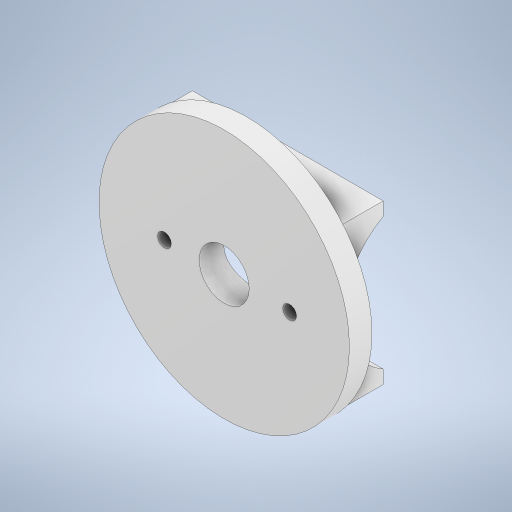
# Autodesk Inventor part: Hub Plate
Saved by Autodesk Inventor 2023 (Build 270158030, 158C)
## iProperties
Created: 2022-10-03
Part Number: Hub Plate
Material: ABS Plastic
Document SubType Name: Modeling
Designer: cjj5381
Density: 1.06 g/cm^3
Appearance: Smooth - White
Author: cjj5381
Autodesk Inventor part; units mm, degrees
ref_plane "YZ Plane" through (0, 0, 0) normal (1, 0, 0) x (0, 1, 0)
ref_plane "XZ Plane" through (0, 0, 0) normal (0, 1, 0) x (-1, 0, 0)
ref_plane "XY Plane" through (0, 0, 0) normal (0, 0, 1) x (1, 0, 0)
sketch "Sketch1" plane through (0, 0, 0) normal (1, 0, 0) x (0, 1, 0)
  circle A0 centre (0, -40) radius 30.1625 construction
  line L0 (31.75, 0) -> (-31.75, 0)
  line L1 (-31.75, 0) -> (-31.75, -25.4)
  line L2 (31.75, -25.4) -> (31.75, 0)
  line L3 (0, 0) -> (0, -115.458)
  arc A1 (26.3935, -25.4) -> (-26.3935, -25.4) centre (0, -40) ccw
  line L4 (-31.75, -25.4) -> (-26.3935, -25.4)
  line L5 (26.3935, -25.4) -> (31.75, -25.4)
  dimension "d1" = 60.325
  dimension "d3" = 63.5
  dimension "d4" = 40
  dimension "d5" = 25.4
  constraints: 12 end point, 4 point on circle, 3 parallel, 2 centre point, 1 concentric, 1 horizontal, 1 midpoint, 1 perpendicular, 1 point on line, 1 vertical, 1 vertical alignment, 1 other
  measures "d1" diameter of A0
  measures "d3" distance of L1.end L2.start
  measures "d4" distance from line of L0 A0.centre
  measures "d5" distance of L0.end L1.end
extrude "Extrusion1" add sketch "Sketch1" along normal mid plane 76.2
sketch "Sketch2" plane through (-38.1, -31.75, 0) normal (0, 0, 1) x (1, 0, 0)
  circle A0 centre (38.1, 31.75) radius 50
  dimension "d8" = 100
  constraints: 1 centre point, 1 coincident
  measures "d8" diameter of A0
extrude "Extrusion2" add sketch "Sketch2" against normal blind 9
sketch "Sketch3" plane through (0, 0, 0) normal (0, 0, 1) x (1, 0, 0)
  circle A0 centre (0, 0) radius 10
  dimension "d11" = 20
  constraints: 1 centre point, 1 coincident
  measures "d11" diameter of A0
extrude "Extrusion3" cut sketch "Sketch3" against normal through all
sketch "Sketch5" plane through (0, 0, 0) normal (0, 0, 1) x (1, 0, 0)
  point P0 (0, 0)
  point P1 (26.1555, 0)
  point P2 (-23.8445, 0)
  point P3 (-23.8445, 0)
  point P4 (26.1555, 0)
  dimension "d23" = 50
  constraints: 2 coincident, 2 horizontal alignment
  measures "d23" distance of point (26.155, 0) point (-23.845, 0)
hole "Hole1" at (26.1555, 0, 0) at (-23.8445, 0, 0) direction (0, 0, -1) diameter 5.5 end through all clearance for "Hex Head Cap Screw ISO 24017" size "M5" standard "ISO"
body "Solid1"
